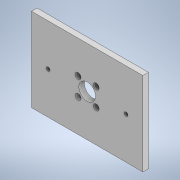
# Autodesk Inventor part: Soporte Piston
Saved by Autodesk Inventor 2021 (Build 250183000, 183)
## iProperties
Created: 2021-05-02
Part Number: Soporte Piston
Material: Generic
Document SubType Name: Modeling
Designer: maaro
Density: 1 g/cm^3
Appearance: Default
Author: maaro
Autodesk Inventor part; units mm, degrees
ref_plane "YZ Plane" through (0, 0, 0) normal (1, 0, 0) x (0, 1, 0)
ref_plane "XZ Plane" through (0, 0, 0) normal (0, 1, 0) x (-1, 0, 0)
ref_plane "XY Plane" through (0, 0, 0) normal (0, 0, 1) x (1, 0, 0)
sketch "Sketch2" plane through (0, 0, 0) normal (0, 0, 1) x (1, 0, 0)
  line L0 (0, 0) -> (200, 0)
  line L1 (200, 0) -> (200, 150)
  line L2 (200, 150) -> (0, 150)
  line L3 (0, 150) -> (0, 0)
  circle A0 centre (100, 75) radius 15
  dimension "d4" = 150
  dimension "d5" = 200
  dimension "d6" = 75
  dimension "d7" = 100
  dimension "d8" = 30
  constraints: 8 end point, 2 parallel, 1 centre point, 1 horizontal, 1 perpendicular
  measures "d4" distance of L2.end L0.start
  measures "d5" distance of L1.end L2.end
  measures "d6" distance from line of A0.centre L2
  measures "d7" distance from line of A0.centre L3
  measures "d8" diameter of A0
extrude "Extrusion2" add sketch "Sketch2" against normal blind 10
sketch "Sketch6" plane through (0, 0, -10) normal (0, 0, -1) x (-1, 0, 0)
  line L0 (0, 150) -> (-200, 150) projected
  line L1 (0, 0) -> (0, 150) projected
  point P0 (-30, 75)
  point P1 (-170, 75)
  dimension "d28" = 75
  dimension "d29" = 75
  dimension "d30" = 140
  dimension "d31" = 30
  measures "d28" distance from line of L0 point (-30, 75)
  measures "d29" distance from line of L0 point (-170, 75)
  measures "d30" distance of point (-170, 75) point (-30, 75)
  measures "d31" distance from line of L1 point (-30, 75)
hole "Hole2" at (30, 75, -10) at (170, 75, -10) direction (0, 0, 1) diameter 6.647 end through all counterbore diameter 14 counterbore depth 5 thread size "M8x1.25" class "6H" standard "ISO Metric profile"
sketch "Sketch7" plane through (0, 0, 0) normal (0, 0, 1) x (1, 0, 0)
  circle A0 centre (83.75, 91.25) radius 3
  circle A1 centre (116.25, 91.25) radius 3
  circle A2 centre (83.75, 58.75) radius 3
  circle A3 centre (116.25, 58.75) radius 3
  circle A4 centre (100, 75) radius 15 projected
  point P0 (0, 0)
  dimension "d39" = 16.25
  dimension "d40" = 16.25
  dimension "d41" = 16.25
  dimension "d42" = 16.25
  dimension "d43" = 16.25
  dimension "d44" = 16.25
  dimension "d45" = 16.25
  dimension "d46" = 16.25
  dimension "d47" = 6
  constraints: 4 centre point, 3 equal radius
  measures "d39" horizontal distance of A2.centre A4.centre
  measures "d40" horizontal distance of A2.centre A4.centre
  measures "d41" horizontal distance of A3.centre A4.centre
  measures "d42" horizontal distance of A3.centre A4.centre
  measures "d43" horizontal distance of A4.centre A0.centre
  measures "d44" horizontal distance of A4.centre A0.centre
  measures "d45" horizontal distance of A4.centre A1.centre
  measures "d46" horizontal distance of A4.centre A1.centre
  measures "d47" diameter of A0
extrude "Extrusion5" cut sketch "Sketch7" against normal blind 15 contours A0 | A1 | A2 | A3
sketch "Sketch8" plane through (0, 0, 0) normal (0, 0, 1) x (1, 0, 0)
  circle A0 centre (83.75, 91.25) radius 3 projected
  circle A1 centre (116.25, 91.25) radius 3 projected
  circle A2 centre (83.75, 58.75) radius 3 projected
  circle A3 centre (116.25, 58.75) radius 3 projected
  circle A4 centre (83.75, 91.25) radius 5.25
  circle A5 centre (116.25, 91.25) radius 5.25
  circle A6 centre (83.75, 58.75) radius 5.25
  circle A7 centre (116.25, 58.75) radius 5.25
  point P0 (0, 0)
  dimension "d50" = 10.5
  dimension "d51" = 10.5
  dimension "d52" = 10.5
  dimension "d53" = 10.5
  constraints: 4 centre point, 4 coincident
  measures "d50" diameter of A4
  measures "d51" diameter of A5
  measures "d52" diameter of A6
  measures "d53" diameter of A7
extrude "Extrusion6" cut sketch "Sketch8" against normal blind 6 contours A0 | A2 | A3 | A4 | A5 | A6 | A7
equation "\"d29\" = d28"
equation "\"d40\" = d39"
equation "\"d41\" = d39"
equation "\"d42\" = d39"
equation "\"d43\" = d39"
equation "\"d44\" = d39"
equation "\"d45\" = d39"
equation "\"d46\" = d39"
equation "\"d50\" = d52"
equation "\"d51\" = d52"
equation "\"d53\" = d52"
body "Solid2"
